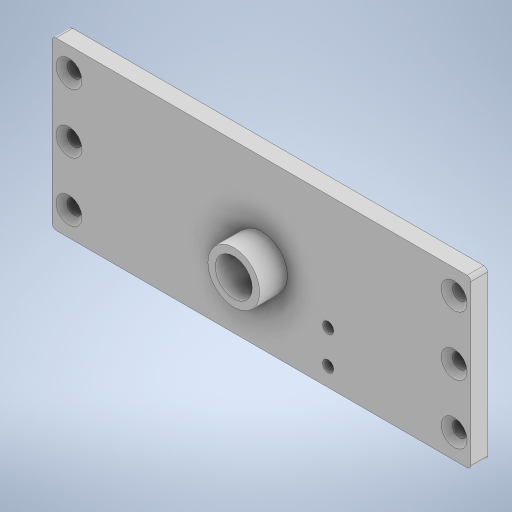
# Autodesk Inventor part: HUDSON 1-05-TRUCK BOLSTER PLATE
Saved by Autodesk Inventor 2024.2 (Build 282272000, 272)
## iProperties
Created: 2024-09-30
Part Number: HUDSON 1-05-TRUCK BOLSTER PLATE
Material: Generic
Document SubType Name: Modeling
Designer: Jimena Brenes
Density: 1 g/cm^3
Appearance: Default
Author: Jimena Brenes
Autodesk Inventor part; units mm, degrees
ref_plane "YZ Plane" through (0, 0, 0) normal (1, 0, 0) x (0, 1, 0)
ref_plane "XZ Plane" through (0, 0, 0) normal (0, 1, 0) x (-1, 0, 0)
ref_plane "XY Plane" through (0, 0, 0) normal (0, 0, 1) x (1, 0, 0)
sketch "Sketch1" plane through (0, 0, 0) normal (0, 0, 1) x (1, 0, 0)
  line L0 (0, 0) -> (113, 0)
  line L1 (113, 0) -> (113, 45)
  line L2 (113, 45) -> (0, 45)
  line L3 (0, 45) -> (0, 0)
  dimension "d0" = 113
  dimension "d1" = 45
  constraints: 8 end point, 2 parallel, 1 horizontal, 1 perpendicular
  measures "d0" distance between parallel lines of L1 L3
  measures "d1" distance between parallel lines of L2 L0
extrude "Extrusion1" add sketch "Sketch1" along normal blind 4.5
sketch "Sketch2" plane through (0, 0, 4.5) normal (0, 0, 1) x (1, 0, 0)
  circle A0 centre (56.5, 20.5) radius 7
  circle A1 centre (56.5, 20.5) radius 5
  line L0 (113, 0) -> (113, 45) projected
  line L1 (0, 0) -> (113, 0) projected
  line L2 (4.5, 38.5) -> (4.5, 6.5) construction
  circle A2 centre (4.5, 38.5) radius 2
  circle A3 centre (4.5, 22.5) radius 2
  circle A4 centre (4.5, 6.5) radius 2
  line L3 (0, 45) -> (0, 0) projected
  line L4 (108.5, 38.5) -> (108.5, 6.5) construction
  circle A5 centre (108.5, 38.5) radius 2
  circle A6 centre (108.5, 22.5) radius 2
  circle A7 centre (108.5, 6.5) radius 2
  line L5 (74.5, 5) -> (74.5, 21.5) construction
  circle A8 centre (74.5, 14) radius 1.5
  circle A9 centre (74.5, 5) radius 1.5
  dimension "d4" = 14
  dimension "d5" = 10
  dimension "d6" = 56.5
  dimension "d7" = 20.5
  dimension "d8" = 4
  dimension "d9" = 4
  dimension "d10" = 4
  dimension "d11" = 4.5
  dimension "d12" = 6.5
  dimension "d13" = 16
  dimension "d14" = 16
  dimension "d15" = 4
  dimension "d16" = 4
  dimension "d17" = 4
  dimension "d18" = 6.5
  dimension "d19" = 16
  dimension "d20" = 16
  dimension "d21" = 4.5
  dimension "d23" = 3
  dimension "d24" = 3
  dimension "d25" = 5
  dimension "d26" = 9
  dimension "d27" = 38.5
  dimension "d51" = 56.5
  constraints: 10 centre point, 6 coincident, 6 end point, 3 midpoint, 3 vertical, 1 point on line
  measures "d4" diameter of A0
  measures "d5" diameter of A1
  measures "d6" distance from line of L0 A0.centre
  measures "d7" distance from line of L1 A0.centre
  measures "d8" diameter of A2
  measures "d9" diameter of A3
  measures "d10" diameter of A4
  measures "d11" distance between parallel lines of L3 L2
  measures "d12" distance from line of L1 L2.end
  measures "d13" distance of A3.centre L2.end
  measures "d14" distance of L2.start A3.centre
  measures "d15" diameter of A5
  measures "d16" diameter of A6
  measures "d17" diameter of A7
  measures "d18" distance from line of L1 L4.end
  measures "d19" distance of point (108.5, 22.5) L4.end
  measures "d20" distance of L4.start A6.centre
  measures "d21" distance from line of L0 L4.end
  measures "d23" diameter of A8
  measures "d24" diameter of A9
  measures "d25" distance from line of L1 L5.start
  measures "d26" distance of A8.centre L5.start
  measures "d27" distance from line of L0 A9.centre
  measures "d51" distance from line of A0.centre L3
extrude "Extrusion2" add sketch "Sketch2" along normal blind 7.5 contours A0
hole "Hole1" at (56.5, 20.5, 4.5) direction (0, 0, -1) diameter 10 end through all
hole "Hole2" at (4.5, 38.5, 4.5) at (4.5, 22.5, 4.5) at (4.5, 6.5, 4.5) at (108.5, 38.5, 4.5) at (108.5, 22.5, 4.5) at (108.5, 6.5, 4.5) direction (0, 0, -1) diameter 4 end through all countersink diameter 7 countersink angle 90
hole "Hole3" at (74.5, 14, 4.5) at (74.5, 5, 4.5) direction (0, 0, -1) diameter 3 end through all
fillet "Fillet1" radius 1 4 edges at (113, 0, 2.25) (113, 45, 2.25) (0, 45, 2.25) (0, 0, 2.25)
body "Solid1"
